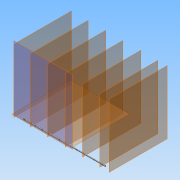
# Autodesk Inventor part: Pancake_Star Shaft 2
Saved by Autodesk Inventor 2018.1 (Build 221171000, 171)
## iProperties
Created: 2019-02-22
Part Number: Pancake_Star Shaft 2
Material: Stainless Steel
Document SubType Name: Modeling
Designer: James
Density: 8 g/cm^3
Appearance: Semi-Polished
Author: James
Autodesk Inventor part; units mm, degrees
ref_plane "YZ Plane" through (0, 0, 0) normal (1, 0, 0) x (0, 1, 0)
ref_plane "XZ Plane" through (0, 0, 0) normal (0, 1, 0) x (-1, 0, 0)
ref_plane "XY Plane" through (0, 0, 0) normal (0, 0, 1) x (1, 0, 0)
derived "Pancake_Skeleton.ipt"
ref_plane "Ground" through (0, 0, 0) normal (0, 1, 0) x (-1, 0, 0)
ref_plane "Back" through (0, 0, 0) normal (0, 0, 1) x (1, 0, 0)
ref_plane "LHS" through (0, 0, 0) normal (1, 0, 0) x (0, 1, 0)
ref_plane "Lane 1" through (90, 0, 0) normal (1, 0, 0) x (0, 1, 0)
ref_plane "Lane 2" through (185, 0, 0) normal (1, 0, 0) x (0, 1, 0)
ref_plane "Lane 3" through (280, 0, 0) normal (1, 0, 0) x (0, 1, 0)
ref_plane "Lane 4" through (375, 0, 0) normal (1, 0, 0) x (0, 1, 0)
ref_plane "Lane 5" through (470, 0, 0) normal (1, 0, 0) x (0, 1, 0)
ref_plane "RHS" through (520, 0, 0) normal (1, 0, 0) x (0, 1, 0)
sketch "Sketch2" plane through (0, 0, 0) normal (0, 0, 1) x (1, 0, 0)
  line L0 (0, 3.6) -> (0, -0.6) projected
  line L1 (90, 3.6) -> (90, -0.6) projected
  line L2 (185, 3.6) -> (185, -0.6) projected
  line L3 (280, 3.6) -> (280, -0.6) projected
  line L4 (375, 3.6) -> (375, -0.6) projected
  line L5 (470, 3.6) -> (470, -0.6) projected
  line L6 (520, 3.6) -> (520, -0.6) projected
  line L7 (-98, 0) -> (588, 0) projected
  line L8 (45, 0) -> (490, 0)
  line L9 (490, 0) -> (490, 3)
  line L10 (490, 3) -> (45, 3)
  line L11 (45, 3) -> (45, 0)
  line L12 (-98, 0) -> (588, 0) projected
  point P0 (0, 0)
  dimension "d1" = 30
  dimension "d2" = 45
  dimension "d3" = 3
  constraints: 8 end point, 2 parallel, 1 horizontal, 1 perpendicular, 1 point on line
  measures "d1" distance between parallel lines of L6 L9
  measures "d2" distance between parallel lines of L0 L11
  measures "d3" distance of L8.end L9.end
revolve "Revolution1" add sketch "Sketch2" angle 360 about axis through (-10, 0, 0) along (1, 0, 0)
sketch "Sketch3" plane through (0, 0, 0) normal (0, 0, 1) x (1, 0, 0)
  line L0 (50.2, 3) -> (51, 3)
  line L1 (51, 3) -> (51, 2.85)
  line L2 (51, 2.85) -> (50.2, 2.85)
  line L3 (50.2, 2.85) -> (50.2, 3)
  line L4 (-10.2, 0) -> (61.2, 0) projected
  line L5 (45, -3) -> (45, 3) projected
  line L6 (90, 4.2) -> (90, -4.2) projected
  line L7 (-10.2, 0) -> (61.2, 0) projected
  line L8 (185, 4.2) -> (185, -4.2) projected
  line L9 (0, 4.2) -> (0, -4.2) projected
  point P0 (0, 0)
  dimension "d5" = 0.8
  dimension "d6" = 2.85
  dimension "d19" = 95
  dimension "d21" = 39
  dimension "d22" = 51
  constraints: 8 end point, 2 parallel, 1 horizontal, 1 horizontal alignment, 1 perpendicular
  measures "d5" distance of L0.start L0.end
  measures "d6" distance between parallel lines of L4 L2
  measures "d19" distance between parallel lines of L8 L6
  measures "d21" distance from line of L6 L0.end
  measures "d22" distance from line of L0.end L9
revolve "Revolution2" cut sketch "Sketch3" angle 360 about axis through (-10, 0, 0) along (1, 0, 0)
pattern_linear "Rectangular Pattern1" count 5 spacing 95 along (1, 0, 0) of "Revolution2"
sketch "Sketch4" plane through (0, 0, 0) normal (0, 0, 1) x (1, 0, 0)
  line L0 (108.8, 3) -> (109.6, 3)
  line L1 (109.6, 3) -> (109.6, 2.85)
  line L2 (109.6, 2.85) -> (108.8, 2.85)
  line L3 (108.8, 2.85) -> (108.8, 3)
  line L4 (45, -3) -> (45, 3) projected
  line L5 (-15.16, 0) -> (90.96, 0) projected
  line L6 (0, 4.2) -> (0, -4.2) projected
  line L7 (-15.16, 0) -> (90.96, 0) projected
  point P0 (0, 0)
  dimension "d14" = 2.85
  dimension "d15" = 0.8
  dimension "d17" = 108.8
  constraints: 8 end point, 2 parallel, 1 horizontal, 1 horizontal alignment, 1 perpendicular
  measures "d14" distance between parallel lines of L2 L5
  measures "d15" distance of L0.start L0.end
  measures "d17" distance from line of L0.start L6
revolve "Revolution3" cut sketch "Sketch4" angle 360 about axis through (-10, 0, 0) along (1, 0, 0)
pattern_linear "Rectangular Pattern2" count 2 spacing 367 along (1, 0, 0) of "Revolution3"
chamfer "Chamfer1" distance 0.5 angle 45 2 edges at (45, -3, 0) (490, -3, 0)
body "Solid1"
